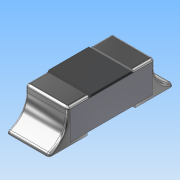
# Autodesk Inventor part: RC0402FR-074K7L Resistor
Saved by Autodesk Inventor 2016 (Build 200138000, 138)
## iProperties
Created: 2019-08-18
Part Number: RC0402FR-074K7L Resistor
Material: Generic
Document SubType Name: Modeling
Designer: Orest
Mass: 0.000219122 g
Surface Area: 0.0264833 cm^2
Volume: 0.000219122 cm^3
Density: 1 g/cm^3
Appearance: White
Author: Orest
Autodesk Inventor part; units mm, degrees
ref_plane "YZ Plane" through (0, 0, 0) normal (1, 0, 0) x (0, 1, 0)
ref_plane "XZ Plane" through (0, 0, 0) normal (0, 1, 0) x (-1, 0, 0)
ref_plane "XY Plane" through (0, 0, 0) normal (0, 0, 1) x (1, 0, 0)
sketch "Sketch10" plane through (0, 0, 0) normal (0, 0, 1) x (1, 0, 0)
  line L0 (-0.485, 0.17) -> (0.485, 0.17)
  line L1 (0.485, 0.17) -> (0.485, -0.17)
  line L2 (0.485, -0.17) -> (-0.485, -0.17)
  line L3 (-0.485, -0.17) -> (-0.485, 0.17)
  line L4 (-0.265, 0.17) -> (-0.485, 0.17)
  line L5 (-0.515, 0.2) -> (-0.265, 0.2)
  line L6 (-0.265, 0.2) -> (-0.265, 0.17)
  line L7 (-0.515, 0.2) -> (-0.515, -0.17)
  line L8 (-0.485, -0.17) -> (-0.485, 0.17)
  line L9 (-0.285, -0.17) -> (-0.285, -0.2)
  line L10 (-0.285, -0.2) -> (-0.735, -0.2)
  line L11 (-0.735, -0.2) -> (-0.735, -0.17)
  line L12 (-0.735, -0.17) -> (-0.515, -0.17)
  line L13 (-0.485, -0.17) -> (-0.285, -0.17)
  line L14 (-0.265, 0.17) -> (0.265, 0.17)
  line L15 (0.265, 0.17) -> (0.235, 0.2)
  line L16 (0.235, 0.2) -> (-0.235, 0.2)
  line L17 (-0.235, 0.2) -> (-0.265, 0.17)
  point P0 (0, 0)
  point P1 (0, 0.17)
  point P2 (-0.485, 0)
  point P3 (0, 0.2)
  dimension "d11" = 0.2
  dimension "d12" = 0.45
  dimension "d13" = 0.03
  dimension "d14" = 0.03
  dimension "d15" = 0.25
  dimension "d16" = 45
  dimension "d19" = 0.03
  dimension "d21" = 1
  dimension "d22" = 0.4
  constraints: 36 end point, 8 parallel, 6 collinear, 5 horizontal, 5 perpendicular, 3 midpoint, 2 vertical alignment, 1 horizontal alignment
  measures "d11" distance from line of L9.end L3
  measures "d12" distance between parallel lines of L9 L11
  measures "d13" distance between parallel lines of L3 L7
  measures "d14" distance between parallel lines of L10 L12
  measures "d15" distance between parallel lines of L6 L7
  measures "d16" angle of L14 L17
  measures "d19" distance between parallel lines of L0 L5
  measures "d21" distance between parallel lines of L1 L7
  measures "d22" distance between parallel lines of L10 L5
extrude "Extrusion4" add sketch "Sketch10" along normal mid plane 0.499 contours L0 L1 L2 L3
extrude "Extrusion5" add sketch "Sketch10" along normal mid plane 0.5 contours L3 L2 L9 L10 L11 L12 L7 L5 L6 L0 | L17 L16 L15 L0
fillet "Fillet2" radius 0.3 1 edges at (-0.515, -0.17, 0)
fillet "Fillet3" radius 0.029 10 edges at (-0.39, 0.2, 0.25) (-0.515, 0.2, 0) (-0.39, 0.2, -0.25) (-0.5763, -0.0625, -0.25) (-0.515, 0.1596, -0.25) (-0.5763, -0.0625, 0.25) (-0.515, 0.1596, 0.25) (-0.735, -0.185, 0.25) (-0.735, -0.17, 0) (-0.735, -0.185, -0.25)
mirror "Mirror1" about plane through (0, 0, 0) normal (1, 0, 0) of "Extrusion5", "Fillet2", "Fillet3"
equation "\"d14\" = d13"
equation "\"d19\" = d13"
body "Solid4"
